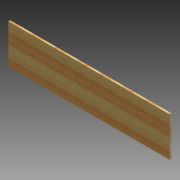
# Autodesk Inventor part: plywood back pannel 2
Saved by Autodesk Inventor 2012 (Build 160160000, 160)
## iProperties
Created: 2013-09-02
Part Number: plywood back pannel 2
Material: Default
Document SubType Name: Modeling
Designer: Bryce
Density: 1 g/cm^3
Author: Bryce
Autodesk Inventor part; units mm, degrees
ref_plane "YZ Plane" through (0, 0, 0) normal (1, 0, 0) x (0, 1, 0)
ref_plane "XZ Plane" through (0, 0, 0) normal (0, 1, 0) x (-1, 0, 0)
ref_plane "XY Plane" through (0, 0, 0) normal (0, 0, 1) x (1, 0, 0)
sketch "Sketch1" plane through (0, 0, 0) normal (0, 0, 1) x (1, 0, 0)
  line L0 (0, 0) -> (939.8, 0)
  line L1 (939.8, 0) -> (939.8, 228.6)
  line L2 (939.8, 228.6) -> (0, 228.6)
  line L3 (0, 228.6) -> (0, 0)
  line L4 (152.4, 88.9) -> (279.4, 88.9) construction
  line L5 (279.4, 88.9) -> (279.4, 215.9) construction
  line L6 (279.4, 215.9) -> (152.4, 215.9) construction
  line L7 (152.4, 215.9) -> (152.4, 88.9) construction
  line L8 (152.4, 88.9) -> (279.4, 215.9) construction
  line L9 (279.4, 88.9) -> (152.4, 215.9) construction
  circle A0 centre (265.9, 202.4) radius 3.175
  circle A1 centre (265.9, 102.4) radius 3.175
  circle A2 centre (165.9, 102.4) radius 3.175
  circle A3 centre (165.9, 202.4) radius 3.175
  line L10 (273.05, 200.5697) -> (273.05, 104.2303)
  line L11 (273.05, 104.2303) -> (224.8803, 152.4)
  line L12 (224.8803, 152.4) -> (273.05, 200.5697)
  line L13 (167.7303, 209.55) -> (264.0697, 209.55)
  line L14 (264.0697, 209.55) -> (215.9, 161.3803)
  line L15 (215.9, 161.3803) -> (167.7303, 209.55)
  line L16 (158.75, 104.2303) -> (158.75, 200.5697)
  line L17 (158.75, 200.5697) -> (206.9197, 152.4)
  line L18 (206.9197, 152.4) -> (158.75, 104.2303)
  line L19 (264.0697, 95.25) -> (167.7303, 95.25)
  line L20 (167.7303, 95.25) -> (215.9, 143.4197)
  line L21 (215.9, 143.4197) -> (264.0697, 95.25)
  line L22 (279.4, 88.9) -> (406.4, 88.9) construction
  line L23 (406.4, 88.9) -> (406.4, 215.9) construction
  line L24 (406.4, 215.9) -> (279.4, 215.9) construction
  line L25 (279.4, 215.9) -> (279.4, 88.9) construction
  line L26 (279.4, 88.9) -> (406.4, 215.9) construction
  line L27 (406.4, 88.9) -> (279.4, 215.9) construction
  circle A4 centre (392.9, 202.4) radius 3.175
  circle A5 centre (392.9, 102.4) radius 3.175
  circle A6 centre (292.9, 102.4) radius 3.175
  circle A7 centre (292.9, 202.4) radius 3.175
  line L28 (400.05, 200.5697) -> (400.05, 104.2303)
  line L29 (400.05, 104.2303) -> (351.8803, 152.4)
  line L30 (351.8803, 152.4) -> (400.05, 200.5697)
  line L31 (294.7303, 209.55) -> (391.0697, 209.55)
  line L32 (391.0697, 209.55) -> (342.9, 161.3803)
  line L33 (342.9, 161.3803) -> (294.7303, 209.55)
  line L34 (285.75, 104.2303) -> (285.75, 200.5697)
  line L35 (285.75, 200.5697) -> (333.9197, 152.4)
  line L36 (333.9197, 152.4) -> (285.75, 104.2303)
  line L37 (391.0697, 95.25) -> (294.7303, 95.25)
  line L38 (294.7303, 95.25) -> (342.9, 143.4197)
  line L39 (342.9, 143.4197) -> (391.0697, 95.25)
  line L40 (406.4, 88.9) -> (533.4, 88.9) construction
  line L41 (533.4, 88.9) -> (533.4, 215.9) construction
  line L42 (533.4, 215.9) -> (406.4, 215.9) construction
  line L43 (406.4, 215.9) -> (406.4, 88.9) construction
  line L44 (406.4, 88.9) -> (533.4, 215.9) construction
  line L45 (533.4, 88.9) -> (406.4, 215.9) construction
  circle A8 centre (519.9, 202.4) radius 3.175
  circle A9 centre (519.9, 102.4) radius 3.175
  circle A10 centre (419.9, 102.4) radius 3.175
  circle A11 centre (419.9, 202.4) radius 3.175
  line L46 (527.05, 200.5697) -> (527.05, 104.2303)
  line L47 (527.05, 104.2303) -> (478.8803, 152.4)
  line L48 (478.8803, 152.4) -> (527.05, 200.5697)
  line L49 (421.7303, 209.55) -> (518.0697, 209.55)
  line L50 (518.0697, 209.55) -> (469.9, 161.3803)
  line L51 (469.9, 161.3803) -> (421.7303, 209.55)
  line L52 (412.75, 104.2303) -> (412.75, 200.5697)
  line L53 (412.75, 200.5697) -> (460.9197, 152.4)
  line L54 (460.9197, 152.4) -> (412.75, 104.2303)
  line L55 (518.0697, 95.25) -> (421.7303, 95.25)
  line L56 (421.7303, 95.25) -> (469.9, 143.4197)
  line L57 (469.9, 143.4197) -> (518.0697, 95.25)
  line L58 (533.4, 88.9) -> (660.4, 88.9) construction
  line L59 (660.4, 88.9) -> (660.4, 215.9) construction
  line L60 (660.4, 215.9) -> (533.4, 215.9) construction
  line L61 (533.4, 215.9) -> (533.4, 88.9) construction
  line L62 (533.4, 88.9) -> (660.4, 215.9) construction
  line L63 (660.4, 88.9) -> (533.4, 215.9) construction
  circle A12 centre (646.9, 202.4) radius 3.175
  circle A13 centre (646.9, 102.4) radius 3.175
  circle A14 centre (546.9, 102.4) radius 3.175
  circle A15 centre (546.9, 202.4) radius 3.175
  line L64 (654.05, 200.5697) -> (654.05, 104.2303)
  line L65 (654.05, 104.2303) -> (605.8803, 152.4)
  line L66 (605.8803, 152.4) -> (654.05, 200.5697)
  line L67 (548.7303, 209.55) -> (645.0697, 209.55)
  line L68 (645.0697, 209.55) -> (596.9, 161.3803)
  line L69 (596.9, 161.3803) -> (548.7303, 209.55)
  line L70 (539.75, 104.2303) -> (539.75, 200.5697)
  line L71 (539.75, 200.5697) -> (587.9197, 152.4)
  line L72 (587.9197, 152.4) -> (539.75, 104.2303)
  line L73 (645.0697, 95.25) -> (548.7303, 95.25)
  line L74 (548.7303, 95.25) -> (596.9, 143.4197)
  line L75 (596.9, 143.4197) -> (645.0697, 95.25)
  line L76 (660.4, 88.9) -> (787.4, 88.9) construction
  line L77 (787.4, 88.9) -> (787.4, 215.9) construction
  line L78 (787.4, 215.9) -> (660.4, 215.9) construction
  line L79 (660.4, 215.9) -> (660.4, 88.9) construction
  line L80 (660.4, 88.9) -> (787.4, 215.9) construction
  line L81 (787.4, 88.9) -> (660.4, 215.9) construction
  circle A16 centre (773.9, 202.4) radius 3.175
  circle A17 centre (773.9, 102.4) radius 3.175
  circle A18 centre (673.9, 102.4) radius 3.175
  circle A19 centre (673.9, 202.4) radius 3.175
  line L82 (781.05, 200.5697) -> (781.05, 104.2303)
  line L83 (781.05, 104.2303) -> (732.8803, 152.4)
  line L84 (732.8803, 152.4) -> (781.05, 200.5697)
  line L85 (675.7303, 209.55) -> (772.0697, 209.55)
  line L86 (772.0697, 209.55) -> (723.9, 161.3803)
  line L87 (723.9, 161.3803) -> (675.7303, 209.55)
  line L88 (666.75, 104.2303) -> (666.75, 200.5697)
  line L89 (666.75, 200.5697) -> (714.9197, 152.4)
  line L90 (714.9197, 152.4) -> (666.75, 104.2303)
  line L91 (772.0697, 95.25) -> (675.7303, 95.25)
  line L92 (675.7303, 95.25) -> (723.9, 143.4197)
  line L93 (723.9, 143.4197) -> (772.0697, 95.25)
  point P0 (215.9, 152.4)
  point P1 (342.9, 152.4)
  point P2 (469.9, 152.4)
  point P3 (596.9, 152.4)
  point P4 (723.9, 152.4)
  dimension "d0" = 939.8
  dimension "d1" = 228.6
  dimension "d4" = 152.4
  dimension "d6" = 127
  dimension "d7" = 127
  dimension "d10" = 12.7
  dimension "d18" = 100
  dimension "d19" = 100
  dimension "d20" = 6.35
  dimension "d21" = 6.35
  dimension "d22" = 6.35
  dimension "d23" = 6.35
  dimension "d26" = 360
  dimension "d30" = 127
  constraints: 188 end point, 20 centre point, 20 point on line, 6 parallel, 3 equal radius, 3 horizontal, 3 perpendicular, 2 vertical alignment, 1 midpoint, 197 other
  measures "d0" distance of L1.end L2.end
  measures "d1" distance of L2.end L0.start
  measures "d4" distance between parallel lines of L3 L7
  measures "d6" distance of L5.end L6.end
  measures "d7" distance of L6.end L4.start
  measures "d10" distance between parallel lines of L2 L6
  measures "d18" distance of A3.centre A0.centre
  measures "d19" distance of A2.centre A3.centre
  measures "d20" diameter of A2
  measures "d21" distance between parallel lines of L5 L10
  measures "d22" distance between parallel lines of L9 L11
  measures "d23" distance from line of L8 L11.end
  measures "d30" distance of L5.end L24.start
extrude "Extrusion1" add sketch "Sketch1" along normal blind 11.1125 contours L3 L2 L1 L0 | A0 | A1 | A2 | A3 | L10 L11 L12 | L13 L14 L15 | L16 L17 L18 | L19 L20 L21 | A4 | A5 | A6 | A7 | L28 L29 L30 | L31 L32 L33 | L34 L35 L36 | L37 L38 L39 | A8 | A9 | A10 | A11 | L46 L47 L48 | L49 L50 L51 | L52 L53 L54 | L55 L56 L57 | A12 | A13 | A14 | A15 | L64 L65 L66 | L67 L68 L69 | L70 L71 L72 | L73 L74 L75 | A16 | A17 | A18 | A19 | L82 L83 L84 | L85 L86 L87 | L88 L89 L90 | L91 L92 L93
fillet "Fillet1" [suppressed]
body "Solid1"
